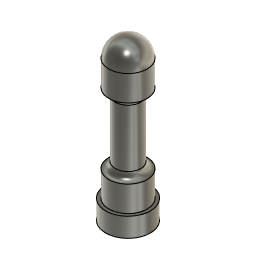
Valve_Lifter v2 (Autodesk Fusion 360 design; units mm, degrees)
Autodesk Fusion 360 part; units mm, degrees
note: some values were not read from the file. Set by a fixed rule: which sketch regions a step uses.
sketch "Sketch1" plane through (0, 0, 0) normal (0, 1, 0) x (1, 0, 0)
  line L0 (5, 0) -> (7, 0)
  line L1 (7, 0) -> (7, -3)
  line L2 (6.5, -3) -> (6.5, -7)
  line L3 (5.5, -17) -> (5.5, -8)
  line L4 (6.5, -18) -> (6.5, -22)
  arc A0 (3.5, -25) -> (6.5, -22) centre (3.5, -22) ccw
  line L5 (0.5, -18) -> (0.5, -18)
  line L6 (6.5, -18) -> (6.5, -18)
  line L7 (6.5, -7) -> (6.5, -7)
  line L8 (0.5, -7) -> (0.5, -7)
  arc A1 (5.5, -17) -> (6.5, -18) centre (6.5, -17) ccw
  arc A2 (6.5, -7) -> (5.5, -8) centre (6.5, -8) ccw
  line L9 (7, -3) -> (6.5, -3)
  line L10 (0.5, -3) -> (0, -3)
  line L11 (3.5, 0) -> (3.5, -25) construction
  line L12 (3.5, -25) -> (3.5, -1.5)
  arc A3 (3.5, -1.5) -> (5, 0) centre (3.5, 0) ccw
  point P0 (5.5, -7)
  point P1 (1.5, -7)
  point P2 (5.5, -18)
  dimension "d10" = 7
  dimension "d11" = 3
  dimension "d12" = 6
  dimension "d13" = 4
  dimension "d14" = 4
  dimension "d15" = 11
  dimension "d16" = 6
  dimension "d17" = 6
  dimension "d18" = 4
  dimension "d20" = 1
  dimension "d22" = 1
  dimension "d25" = 3
  constraint horizontal L0
  constraint vertical L1
  constraint horizontal L9
  constraint vertical L2
  constraint coincident L10.start L9
  constraint vertical L3
  constraint vertical L4
  constraint coincident P2 L3
  constraint coincident P2 L6
  constraint tangent L3 A1
  constraint coincident P1 L8
  constraint coincident P0 L3
  constraint coincident P0 L7
  constraint tangent L3 A2
  constraint collinear L9 L10
  constraint coincident L11.start A3.centre
  constraint coincident L11 L12.end
  measures "d10" distance of origin L0.end
  measures "d11" distance of origin L10.end
  measures "d12" distance of L10.start L2.start
  measures "d13" distance of L2.start L2.end
  measures "d14" distance of P0 P1
  measures "d15" distance of P0 P2
  measures "d16" distance of L5.start L4.start
  measures "d17" diameter of A0
  measures "d18" distance of L4.start L4.end
  measures "d20" radius of A1
  measures "d22" radius of A2
  measures "d25" diameter of A3
revolve "Revolve1" add sketch "Sketch1" angle 360 about axis through (3.5, 0, 25) along (0, 0, -1)
equation "lifter_tier_one_height = 3 mm"
equation "lifter_tier_one_diameter = 7 mm"
equation "lifter_tier_two_height = 4 mm"
equation "lifter_tier_two_diameter = 6 mm"
equation "lifter_tier_three_height = 11 mm"
equation "lifter_tier_three_diameter = 4 mm"
equation "lifter_tier_three_radius = 1 mm"
equation "lifter_tier_four_diameter = 6 mm"
equation "lifter_tier_four_total_height = 7 mm"
equation "d10 = lifter_tier_one_diameter"
equation "d11 = lifter_tier_one_height"
equation "d12 = lifter_tier_two_diameter"
equation "d13 = lifter_tier_two_height"
equation "d14 = lifter_tier_three_diameter"
equation "d15 = lifter_tier_three_height"
equation "d16 = lifter_tier_four_diameter"
equation "d17 = lifter_tier_four_diameter"
equation "d18 = lifter_tier_four_total_height - ( lifter_tier_four_diameter / 2 )"
equation "d20 = lifter_tier_three_radius"
equation "d22 = lifter_tier_three_radius"
equation "hemispherical_cut_diameter = 3 mm"
equation "d25 = hemispherical_cut_diameter"
